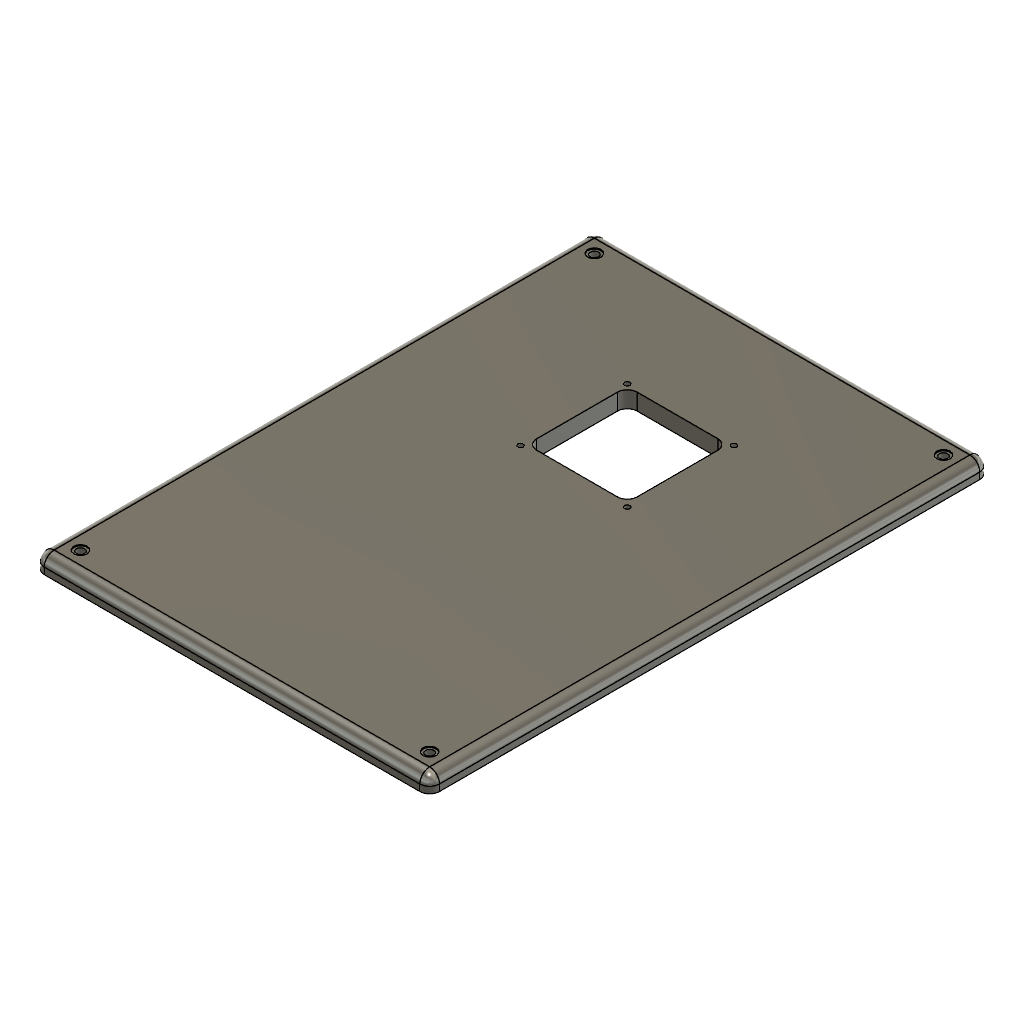
DMX Unit up (Autodesk Fusion 360 design; units mm, degrees)
part number: 2026-09-09-19-26-09-695
Autodesk Fusion 360 part; units mm, degrees
note: some values were not read from the file. Chosen so that the rebuilt part matches the saved one: which face or edge a step refers to; a direction.
(part 1 of 2)
sketch "Esquisse1" plane through (0, 0, 0) normal (0, 1, 0) x (1, 0, 0)
  line L0 (0, 0) -> (120, 0)
  line L1 (120, 0) -> (120, 170)
  line L2 (120, 170) -> (0, 170)
  line L3 (0, 170) -> (0, 0)
  dimension "d1" = 120
  dimension "d2" = 170
  constraint horizontal L0
  constraint vertical L1
  constraint horizontal L2
  constraint vertical L3
  constraint coincident L0.start L3.end
  measures "d1" distance of L0.start L0.end
  measures "d2" distance of L0.end L1.end
sketch "Esquisse2" plane through (0, 100, 0) normal (0, 1, 0) x (1, 0, 0)
  line L0 (5, 165) -> (115, 165)
  line L1 (115, 165) -> (115, 5)
  line L2 (115, 5) -> (5, 5)
  line L3 (5, 5) -> (5, 165)
  line L4 (0, 170) -> (120, 170)
  line L5 (120, 170) -> (120, 0)
  line L6 (120, 0) -> (0, 0)
  line L7 (0, 0) -> (0, 170)
  line L8 (0, 170) -> (0, 0)
  line L9 (0, 0) -> (120, 0)
  line L10 (120, 0) -> (120, 170)
  line L11 (120, 170) -> (0, 170)
  dimension "d5" = 120
  dimension "d6" = 170
  dimension "d7" = 5
  dimension "d8" = 5
  dimension "d9" = 5
  dimension "d10" = 5
  constraint horizontal L0
  constraint vertical L1
  constraint vertical L3
  constraint horizontal L4
  constraint vertical L5
  constraint horizontal L6
  constraint vertical L7
  measures "d5" distance of L4.start L4.end
  measures "d6" distance of L4.end L5.end
  measures "d7" distance of L0 L4
  measures "d8" distance of L3 L7
  measures "d9" distance of L2 L6
  measures "d10" distance of L1 L5
sketch "Esquisse3" plane through (0, 0, 0) normal (0, 0, 1) x (1, 0, 0)
  line L0 (0, 0) -> (120, 0)
  line L1 (120, 0) -> (120, 100)
  line L2 (120, 100) -> (0, 100)
  line L3 (0, 100) -> (0, 0)
  line L4 (0, 100) -> (120, 100)
  line L5 (120, 100) -> (120, 0)
  line L6 (120, 0) -> (0, 0)
  line L7 (0, 0) -> (0, 100)
  circle A0 centre (30, 30) radius 8
  circle A1 centre (90, 30) radius 8
  line L8 (52, 70) -> (68, 70)
  line L9 (68, 70) -> (68, 57)
  line L10 (68, 57) -> (52, 57)
  line L11 (52, 57) -> (52, 70)
  dimension "d13" = 16
  dimension "d14" = 30
  dimension "d15" = 120
  dimension "d16" = 30
  dimension "d17" = 16
  dimension "d18" = 30
  dimension "d19" = 30
  dimension "d20" = 16
  dimension "d21" = 13
  dimension "d22" = 52
  constraint horizontal L4
  constraint vertical L5
  constraint horizontal L6
  constraint vertical L7
  constraint coincident L2.end L3.start
  constraint horizontal L8
  constraint vertical L9
  constraint horizontal L10
  constraint vertical L11
  measures "d13" diameter of A0
  measures "d14" distance of L6 A0.centre
  measures "d15" distance of L0.end L0.start
  measures "d16" distance of L7 A0.centre
  measures "d17" diameter of A1
  measures "d18" distance of L6 A1.centre
  measures "d19" distance of L5 A1.centre
  measures "d20" distance of L8.start L8.end
  measures "d21" distance of L8.end L9.end
  measures "d22" distance of L5 L9
sketch "Esquisse4" plane through (0, 0, 0) normal (0, 0, 1) x (1, 0, 0)
  line L0 (68, 70) -> (68, 57)
  line L1 (68, 57) -> (52, 57)
  line L2 (52, 57) -> (52, 70)
  line L3 (52, 70) -> (68, 70)
  circle A0 centre (30, 30) radius 8
  circle A1 centre (90, 30) radius 8
  line L4 (0, 0) -> (120, 0)
  line L5 (120, 0) -> (120, 100)
  line L6 (120, 100) -> (0, 100)
  line L7 (0, 100) -> (0, 0)
  line L8 (30, 80) -> (90, 80) construction
  line L9 (90, 80) -> (90, 90) construction
  line L10 (90, 90) -> (30, 90) construction
  line L11 (30, 90) -> (30, 80) construction
  dimension "d25" = 10
sketch "Esquisse5" plane through (0, 0, -170) normal (0, 0, -1) x (-1, 0, 0)
  line L0 (-120, 0) -> (0, 0)
  line L1 (0, 0) -> (0, 100)
  line L2 (0, 100) -> (-120, 100)
  line L3 (-120, 100) -> (-120, 0)
  line L4 (-73, 30) -> (-47, 30)
  line L5 (-47, 30) -> (-47, 20)
  line L6 (-47, 20) -> (-73, 20)
  line L7 (-73, 20) -> (-73, 30)
  dimension "d29" = 26
  dimension "d30" = 10
  dimension "d31" = 20
  dimension "d32" = 47
  constraint horizontal L4
  constraint vertical L5
  constraint horizontal L6
  constraint vertical L7
  measures "d29" distance of L4.start L4.end
  measures "d30" distance of L4.end L5.end
  measures "d31" distance of L0 L6
  measures "d32" distance of L1 L5
sketch "Esquisse6" plane through (0, 0, -170) normal (0, 0, -1) x (-1, 0, 0)
  line L0 (-120, 0) -> (0, 0)
  line L1 (0, 0) -> (0, 100)
  line L2 (0, 100) -> (-120, 100)
  line L3 (-120, 100) -> (-120, 0)
  line L4 (-90, 70) -> (-30, 70) construction
  line L5 (-30, 70) -> (-30, 80) construction
  line L6 (-30, 80) -> (-90, 80) construction
  line L7 (-90, 80) -> (-90, 70) construction
  dimension "d35" = 10
sketch "Esquisse7" plane through (0, 0, 0) normal (0, 1, 0) x (1, 0, 0)
  line L0 (-50, 0) -> (-170, 0)
  line L1 (-170, 0) -> (-170, 170)
  line L2 (-170, 170) -> (-50, 170)
  line L3 (-50, 170) -> (-50, 0)
  constraint horizontal L0
  constraint vertical L1
  constraint horizontal L2
  constraint vertical L3
extrude "Extrusion7" add sketch "Esquisse7" along normal blind 5
sketch "Esquisse8" plane through (0, 5, 0) normal (0, 1, 0) x (-1, 0, 0)
  line L0 (50, -170) -> (170, -170)
  line L1 (170, -170) -> (170, 0)
  line L2 (170, 0) -> (50, 0)
  line L3 (50, 0) -> (50, -170)
  line L4 (90, -100) -> (125, -100)
  line L5 (125, -100) -> (125, -135)
  line L6 (125, -135) -> (90, -135)
  line L7 (90, -135) -> (90, -100)
  line L8 (50, 0) -> (170, 0)
  line L9 (170, 0) -> (170, -170)
  line L10 (170, -170) -> (50, -170)
  line L11 (50, -170) -> (50, 0)
  dimension "d41" = 35
  dimension "d42" = 35
  dimension "d43" = 45
  dimension "d44" = 35
  dimension "d45" = 170
  dimension "d46" = 120
  constraint horizontal L4
  constraint vertical L5
  constraint horizontal L6
  constraint vertical L7
  constraint horizontal L8
  constraint vertical L9
  constraint horizontal L10
  constraint vertical L11
  constraint coincident L0.end L1.start
  constraint coincident L2.end L3.start
  measures "d41" distance of L4.start L4.end
  measures "d42" distance of L4.end L5.end
  measures "d43" distance of L1 L5
  measures "d44" distance of L0 L6
  measures "d45" distance of L1.end L0.end
  measures "d46" distance of L2.end L1.end
extrude "Extrusion8" cut sketch "Esquisse8" against normal blind 60 contours L4 L5 L6 L7
fillet "Congé3" radius 3 4 edges at (-110, 5, 0) (-50, 5, -85) (-170, 5, -85) (-110, 5, -170)
sketch "Esquisse9" plane through (0, 0, 0) normal (0, 0, 1) x (1, 0, 0)
  line L0 (117, 3) -> (117, 100)
  line L1 (3, 100) -> (3, 3)
  line L2 (3, 3) -> (117, 3)
  spline S0 degree 3 poles (27.9161, 84.9932) (27.9562, 85.7465) (28.0314, 87.1592) (28.8829, 88.2822) (29.2804, 88.8063) knots 0 0 0 0 0.220424 0.413335 0.413335 0.413335 0.413335
  spline S1 degree 3 poles (29.2804, 88.8063) (29.8033, 89.2037) (30.9218, 90.0539) (32.3299, 90.13) (33.0798, 90.1705) knots 0 0 0 0 0.192622 0.412035 0.412035 0.412035 0.412035
  spline S2 degree 3 poles (33.0798, 90.1705) (33.8439, 90.1336) (35.2646, 90.0651) (36.4015, 89.2205) (36.927, 88.8301) knots 0 0 0 0 0.223535 0.415648 0.415648 0.415648 0.415648
  spline S3 degree 3 poles (36.927, 88.8301) (37.3205, 88.3148) (38.1635, 87.2105) (38.2379, 85.8178) (38.2776, 85.075) knots 0 0 0 0 0.190128 0.407383 0.407383 0.407383 0.407383
  spline S4 degree 3 poles (38.2776, 85.075) (38.2624, 84.5359) (38.2344, 83.5411) (37.8594, 82.6212) (37.6876, 82.1999) knots 0 0 0 0 0.160213 0.295632 0.295632 0.295632 0.295632
  spline S5 degree 3 poles (37.6876, 82.1999) (37.4686, 81.8464) (37.0298, 81.1378) (36.3319, 80.682) (35.9823, 80.4536) knots 0 0 0 0 0.123109 0.246747 0.246747 0.246747 0.246747
  spline S6 degree 3 poles (35.9823, 80.4536) (35.5708, 80.2718) (34.6869, 79.8813) (33.7196, 79.8475) (33.2026, 79.8295) knots 0 0 0 0 0.133717 0.287224 0.287224 0.287224 0.287224
  spline S7 degree 3 poles (33.2026, 79.8295) (32.6811, 79.8436) (31.7167, 79.8698) (30.8161, 80.2115) (30.4025, 80.3683) knots 0 0 0 0 0.155173 0.28695 0.28695 0.28695 0.28695
  spline S8 degree 3 poles (30.4025, 80.3683) (30.0477, 80.5788) (29.3199, 81.0106) (28.8473, 81.7134) (28.605, 82.0737) knots 0 0 0 0 0.122118 0.250545 0.250545 0.250545 0.250545
  spline S9 degree 3 poles (28.605, 82.0737) (28.4043, 82.5044) (27.9739, 83.4282) (27.9362, 84.4485) (27.9161, 84.9932) knots 0 0 0 0 0.14111 0.302672 0.302672 0.302672 0.302672
  line L3 (61.6542, 90) -> (66.7906, 90)
  spline S10 degree 3 poles (66.7906, 90) (67.2965, 89.9827) (68.214, 89.9514) (68.9666, 89.4341) (69.3042, 89.2019) knots 0 0 0 0 0.148093 0.268627 0.268627 0.268627 0.268627
  spline S11 degree 3 poles (69.3042, 89.2019) (69.5476, 88.8929) (70.0702, 88.2295) (70.1156, 87.3827) (70.1398, 86.9304) knots 0 0 0 0 0.115225 0.247344 0.247344 0.247344 0.247344
  spline S12 degree 3 poles (70.1398, 86.9304) (70.1109, 86.4621) (70.0561, 85.574) (69.4946, 84.8878) (69.2292, 84.5634) knots 0 0 0 0 0.136799 0.259393 0.259393 0.259393 0.259393
  spline S13 degree 3 poles (69.2292, 84.5634) (68.8572, 84.3155) (68.0209, 83.7581) (67.0105, 83.7277) (66.4495, 83.7108) knots 0 0 0 0 0.131606 0.295937 0.295937 0.295937 0.295937
  line L4 (66.4495, 83.7108) -> (64.7578, 83.7108)
  line L5 (64.7578, 83.7108) -> (64.7578, 80)
  line L6 (64.7578, 80) -> (61.6542, 80)
  line L7 (61.6542, 80) -> (61.6542, 90)
  line L8 (78.264, 90) -> (81.3472, 90)
  line L9 (81.3472, 90) -> (81.3472, 84.0421)
  spline S14 degree 3 poles (81.3472, 84.0421) (81.3364, 83.753) (81.3152, 83.1834) (81.1515, 82.6375) (81.0709, 82.3687) knots 0 0 0 0 0.086419 0.170224 0.170224 0.170224 0.170224
  spline S15 degree 3 poles (81.0709, 82.3687) (80.9658, 82.1145) (80.7555, 81.6061) (80.3883, 81.1965) (80.2046, 80.9917) knots 0 0 0 0 0.081874 0.163736 0.163736 0.163736 0.163736
  spline S16 degree 3 poles (80.2046, 80.9917) (80.0113, 80.812) (79.6427, 80.4693) (79.1845, 80.2621) (78.9666, 80.1635) knots 0 0 0 0 0.078572 0.149835 0.149835 0.149835 0.149835
  spline S17 degree 3 poles (78.9666, 80.1635) (78.6385, 80.0662) (77.9335, 79.8571) (77.1977, 79.8391) (76.8042, 79.8295) knots 0 0 0 0 0.102197 0.21965 0.21965 0.21965 0.21965
  spline S18 degree 3 poles (76.8042, 79.8295) (76.5496, 79.8344) (76.0172, 79.8448) (75.4877, 79.9019) (75.2115, 79.9317) knots 0 0 0 0 0.076356 0.159674 0.159674 0.159674 0.159674
  spline S19 degree 3 poles (75.2115, 79.9317) (74.9438, 79.9701) (74.4446, 80.0416) (73.9829, 80.2436) (73.7688, 80.3373) knots 0 0 0 0 0.080667 0.150474 0.150474 0.150474 0.150474
  spline S20 degree 3 poles (73.7688, 80.3373) (73.5773, 80.4518) (73.1823, 80.688) (72.8693, 81.0256) (72.7081, 81.1996) knots 0 0 0 0 0.066557 0.13732 0.13732 0.13732 0.13732
  spline S21 degree 3 poles (72.7081, 81.1996) (72.5619, 81.3825) (72.2822, 81.7325) (72.1249, 82.1515) (72.0498, 82.3516) knots 0 0 0 0 0.069719 0.13342 0.13342 0.13342 0.13342
  spline S22 degree 3 poles (72.0498, 82.3516) (71.9664, 82.6496) (71.8114, 83.2034) (71.7785, 83.7772) (71.7633, 84.0421) knots 0 0 0 0 0.09251 0.171904 0.171904 0.171904 0.171904
  line L10 (71.7633, 84.0421) -> (71.7633, 90)
  line L11 (71.7633, 90) -> (74.8465, 90)
  line L12 (74.8465, 90) -> (74.8465, 83.9003)
  spline S23 degree 3 poles (74.8465, 83.9003) (74.8599, 83.6484) (74.8851, 83.1758) (75.168, 82.7986) (75.3001, 82.6224) knots 0 0 0 0 0.073721 0.138349 0.138349 0.138349 0.138349
  spline S24 degree 3 poles (75.3001, 82.6224) (75.4734, 82.4883) (75.8426, 82.2027) (76.3104, 82.1763) (76.5587, 82.1623) knots 0 0 0 0 0.064202 0.136827 0.136827 0.136827 0.136827
  spline S25 degree 3 poles (76.5587, 82.1623) (76.805, 82.1762) (77.2693, 82.2022) (77.6375, 82.4835) (77.8104, 82.6156) knots 0 0 0 0 0.072093 0.135879 0.135879 0.135879 0.135879
  spline S26 degree 3 poles (77.8104, 82.6156) (77.9425, 82.7913) (78.2274, 83.1701) (78.2512, 83.6454) (78.264, 83.9003) knots 0 0 0 0 0.064484 0.139042 0.139042 0.139042 0.139042
  line L13 (78.264, 83.9003) -> (78.264, 90)
  line L14 (82.691, 90) -> (92.0839, 90)
  line L15 (92.0839, 90) -> (92.0839, 87.5307)
  line L16 (92.0839, 87.5307) -> (88.9325, 87.5307)
  line L17 (88.9325, 87.5307) -> (88.9325, 80)
  line L18 (88.9325, 80) -> (85.8424, 80)
  line L19 (85.8424, 80) -> (85.8424, 87.5307)
  line L20 (85.8424, 87.5307) -> (82.691, 87.5307)
  line L21 (82.691, 87.5307) -> (82.691, 90)
  line L22 (46.4495, 90) -> (49.5327, 90)
  line L23 (49.5327, 90) -> (49.5327, 84.0421)
  spline S27 degree 3 poles (49.5327, 84.0421) (49.522, 83.753) (49.5007, 83.1834) (49.3371, 82.6375) (49.2565, 82.3687) knots 0 0 0 0 0.086419 0.170223 0.170223 0.170223 0.170223
  spline S28 degree 3 poles (49.2565, 82.3687) (49.1513, 82.1145) (48.941, 81.6061) (48.5738, 81.1965) (48.3902, 80.9917) knots 0 0 0 0 0.081874 0.163737 0.163737 0.163737 0.163737
  spline S29 degree 3 poles (48.3902, 80.9917) (48.1969, 80.812) (47.8283, 80.4693) (47.37, 80.2621) (47.1521, 80.1635) knots 0 0 0 0 0.078572 0.149834 0.149834 0.149834 0.149834
  spline S30 degree 3 poles (47.1521, 80.1635) (46.8241, 80.0662) (46.119, 79.8571) (45.3832, 79.8391) (44.9898, 79.8295) knots 0 0 0 0 0.102197 0.21965 0.21965 0.21965 0.21965
  spline S31 degree 3 poles (44.9898, 79.8295) (44.7352, 79.8344) (44.2028, 79.8448) (43.6733, 79.9019) (43.397, 79.9317) knots 0 0 0 0 0.076356 0.159673 0.159673 0.159673 0.159673
  spline S32 degree 3 poles (43.397, 79.9317) (43.1294, 79.9701) (42.6301, 80.0416) (42.1685, 80.2436) (41.9543, 80.3373) knots 0 0 0 0 0.080667 0.150474 0.150474 0.150474 0.150474
  spline S33 degree 3 poles (41.9543, 80.3373) (41.7628, 80.4518) (41.3678, 80.688) (41.0549, 81.0256) (40.8936, 81.1996) knots 0 0 0 0 0.066557 0.13732 0.13732 0.13732 0.13732
  spline S34 degree 3 poles (40.8936, 81.1996) (40.7474, 81.3825) (40.4678, 81.7325) (40.3105, 82.1515) (40.2353, 82.3516) knots 0 0 0 0 0.069719 0.13342 0.13342 0.13342 0.13342
  spline S35 degree 3 poles (40.2353, 82.3516) (40.1519, 82.6496) (39.9969, 83.2034) (39.964, 83.7772) (39.9488, 84.0421) knots 0 0 0 0 0.09251 0.171904 0.171904 0.171904 0.171904
  line L24 (39.9488, 84.0421) -> (39.9488, 90)
  line L25 (39.9488, 90) -> (43.0321, 90)
  line L26 (43.0321, 90) -> (43.0321, 83.9003)
  spline S36 degree 3 poles (43.0321, 83.9003) (43.0455, 83.6484) (43.0706, 83.1758) (43.3535, 82.7986) (43.4857, 82.6224) knots 0 0 0 0 0.073721 0.138349 0.138349 0.138349 0.138349
  spline S37 degree 3 poles (43.4857, 82.6224) (43.6589, 82.4883) (44.0281, 82.2027) (44.4959, 82.1763) (44.7442, 82.1623) knots 0 0 0 0 0.064202 0.136827 0.136827 0.136827 0.136827
  spline S38 degree 3 poles (44.7442, 82.1623) (44.9905, 82.1762) (45.4548, 82.2022) (45.8231, 82.4835) (45.9959, 82.6156) knots 0 0 0 0 0.072093 0.135879 0.135879 0.135879 0.135879
  spline S39 degree 3 poles (45.9959, 82.6156) (46.128, 82.7913) (46.4129, 83.1701) (46.4367, 83.6454) (46.4495, 83.9003) knots 0 0 0 0 0.064484 0.139042 0.139042 0.139042 0.139042
  line L27 (46.4495, 83.9003) -> (46.4495, 90)
  line L28 (50.8765, 90) -> (60.2694, 90)
  line L29 (60.2694, 90) -> (60.2694, 87.5307)
  line L30 (60.2694, 87.5307) -> (57.118, 87.5307)
  line L31 (57.118, 87.5307) -> (57.118, 80)
  line L32 (57.118, 80) -> (54.028, 80)
  line L33 (54.028, 80) -> (54.028, 87.5307)
  line L34 (54.028, 87.5307) -> (50.8765, 87.5307)
  line L35 (50.8765, 87.5307) -> (50.8765, 90)
  line L36 (3, 100) -> (117, 100)
  line L37 (117, 100) -> (117, 3)
  line L38 (117, 3) -> (3, 3)
  line L39 (3, 3) -> (3, 100)
  circle A0 centre (33, 28) radius 12
  circle A1 centre (87, 28) radius 12
  line L40 (42.5, 28) -> (23.5, 28) construction
  line L41 (60, 131) -> (60, -75) construction
  line L42 (23.5, 16) -> (23.5, 40) construction
  circle A2 centre (23.5, 40) radius 1.75
  line L43 (23.5, 28) -> (42.5, 28) construction
  line L44 (42.5, 40) -> (42.5, 16) construction
  circle A3 centre (42.5, 16) radius 1.75
  line L45 (96.5, 28) -> (77.5, 28) construction
  line L46 (77.5, 16) -> (77.5, 40) construction
  circle A4 centre (77.5, 40) radius 1.75
  line L47 (96.5, 40) -> (96.5, 16) construction
  circle A5 centre (96.5, 16) radius 1.75
  line L48 (117, 100) -> (3, 100)
  line L49 (51.95, 57) -> (68.05, 57)
  line L50 (68.05, 57) -> (68.05, 70.5)
  line L51 (68.05, 70.5) -> (51.95, 70.5)
  line L52 (51.95, 70.5) -> (51.95, 57)
  point P0 (33, 28)
  point P1 (33, 28)
  point P2 (33, 28)
  point P3 (87, 28)
  dimension "d55" = 114
  dimension "d56" = 97
  dimension "d59" = 24
  dimension "d60" = 24
  dimension "d61" = 25
  dimension "d62" = 25
  dimension "d63" = 30
  dimension "d64" = 30
  dimension "d69" = 19
  dimension "d70" = 24
  dimension "d71" = 3.5
  dimension "d72" = 19
  dimension "d73" = 24
  dimension "d74" = 3.5
  dimension "d75" = 19
  dimension "d76" = 24
  dimension "d77" = 3.5
  dimension "d78" = 24
  dimension "d79" = 3.5
  dimension "d134" = 13.5
  dimension "d135" = 16.1
  dimension "d136" = 48.95
  dimension "d137" = 48.95
  constraint horizontal L36
  constraint vertical L37
  constraint horizontal L38
  constraint vertical L39
  constraint coincident L0.start L2.end
  constraint coincident L1.start L36.start
  constraint midpoint L40 P2
  constraint coincident P2 P1
  constraint perpendicular L39 L40
  constraint perpendicular L2 L41
  constraint midpoint L40.end L42
  constraint perpendicular L40 L42
  constraint coincident L42.end A2.centre
  constraint midpoint L43 P2
  constraint parallel L40 L43
  constraint midpoint L40.start L44
  constraint perpendicular L43 L44
  constraint coincident L44.end A3.centre
  constraint midpoint L45 P3
  constraint coincident P3 A1.centre
  constraint horizontal L45
  constraint midpoint L45.end L46
  constraint perpendicular L45 L46
  constraint coincident L46.end A4.centre
  constraint midpoint L45.start L47
  constraint perpendicular L45 L47
  constraint coincident L47.end A5.centre
  constraint horizontal L49
  constraint vertical L50
  constraint horizontal L51
  constraint vertical L52
  measures "d55" distance of L1.start L0.end
  measures "d56" distance of L0.end L0.start
  measures "d59" diameter of A0
  measures "d60" diameter of A1
  measures "d61" distance of L38 P3
  measures "d62" distance of L38 P2
  measures "d63" distance of L37 P3
  measures "d64" distance of L39 P2
  measures "d69" distance of L40.start L40.end
  measures "d70" distance of L42.start L42.end
  measures "d71" diameter of A2
  measures "d72" distance of L40.end L40.start
  measures "d73" distance of L44.start L44.end
  measures "d74" diameter of A3
  measures "d75" distance of L45.start L45.end
  measures "d76" distance of L46.start L46.end
  measures "d77" diameter of A4
  measures "d78" distance of L47.start L47.end
  measures "d79" diameter of A5
  measures "d134" distance of L49.start L51.end
  measures "d135" distance of L49.start L49.end
  measures "d136" distance of L37 L50
  measures "d137" distance of L39 L52
extrude "Extrusion9" cut sketch "Esquisse9" against normal blind 20 contours A0 | A1 | A2 | A3 | A4 | A5
sketch "Esquisse10" plane through (0, 0, 0) normal (0, 1, 0) x (1, 0, 0)
sketch "Esquisse11" plane through (0, 10, 0) normal (0, 1, 0) x (-1, 0, 0)
  line L0 (-5, -5) -> (-115, -5)
  line L1 (-115, -5) -> (-115, -165)
  line L2 (-115, -165) -> (-5, -165)
  line L3 (-5, -165) -> (-5, -5)
  line L4 (-5, -165) -> (-13, -165)
  line L5 (-13, -165) -> (-13, -157)
  line L6 (-13, -157) -> (-5, -157)
  line L7 (-5, -157) -> (-5, -165)
  line L8 (-115, -165) -> (-107, -165)
  line L9 (-107, -165) -> (-107, -157)
  line L10 (-107, -157) -> (-115, -157)
  line L11 (-115, -157) -> (-115, -165)
  line L12 (-115, -5) -> (-107, -5)
  line L13 (-107, -5) -> (-107, -13)
  line L14 (-107, -13) -> (-115, -13)
  line L15 (-115, -13) -> (-115, -5)
  line L16 (-5, -5) -> (-13, -5)
  line L17 (-13, -5) -> (-13, -13)
  line L18 (-13, -13) -> (-5, -13)
  line L19 (-5, -13) -> (-5, -5)
  constraint horizontal L4
  constraint vertical L5
  constraint horizontal L6
  constraint vertical L7
  constraint coincident L2.end L3.start
  constraint horizontal L8
  constraint vertical L9
  constraint horizontal L10
  constraint vertical L11
  constraint coincident L1.end L2.start
  constraint horizontal L12
  constraint vertical L13
  constraint horizontal L14
  constraint vertical L15
  constraint coincident L0.end L1.start
  constraint horizontal L16
  constraint vertical L17
  constraint horizontal L18
  constraint vertical L19
  constraint coincident L0.start L3.end
sketch "Esquisse12" plane through (0, 5, 0) normal (0, 1, 0) x (-1, 0, 0)
  line L0 (125, -100) -> (125, -135)
  line L1 (125, -135) -> (90, -135)
  line L2 (90, -135) -> (90, -100)
  line L3 (90, -100) -> (125, -100)
  line L4 (53, -167) -> (167, -167)
  line L5 (167, -167) -> (167, -3)
  line L6 (167, -3) -> (53, -3)
  line L7 (53, -3) -> (53, -167)
  circle A0 centre (163, -163) radius 1.25
  circle A1 centre (57, -163) radius 1.25
  circle A2 centre (57, -7) radius 1.25
  circle A3 centre (163, -7) radius 1.25
  dimension "d86" = 2.5
  dimension "d87" = 4
  dimension "d88" = 4
  dimension "d89" = 2.5
  dimension "d90" = 4
  dimension "d91" = 4
  dimension "d92" = 2.5
  dimension "d93" = 2.5
  dimension "d94" = 4
  dimension "d95" = 4
  dimension "d96" = 4
  dimension "d97" = 4
  measures "d86" diameter of A0
  measures "d87" distance of L4 A0.centre
  measures "d88" distance of L5 A0.centre
  measures "d89" diameter of A1
  measures "d90" distance of L4 A1.centre
  measures "d91" distance of L7 A1.centre
  measures "d92" diameter of A3
  measures "d93" diameter of A2
  measures "d94" distance of L7 A2.centre
  measures "d95" distance of L6 A2.centre
  measures "d96" distance of L6 A3.centre
  measures "d97" distance of L5 A3.centre
extrude "Extrusion11" cut sketch "Esquisse12" against normal blind 60 contours A0 | A1 | A2 | A3
sketch "Esquisse13" plane through (0, 0, -165) normal (0, 0, 1) x (1, 0, 0)
  line L0 (13, 100) -> (13, 10)
  line L1 (13, 10) -> (107, 10)
  line L2 (107, 10) -> (107, 100)
  line L3 (107, 100) -> (13, 100)
sketch "Esquisse14" plane through (0, 0, -170) normal (0, 0, -1) x (-1, 0, 0)
  line L0 (-66.7462, 80) -> (-61.6098, 80)
  spline S0 degree 3 poles (-61.6098, 80) (-61.104, 79.9827) (-60.1864, 79.9514) (-59.4338, 79.4341) (-59.0962, 79.2019) knots 0 0 0 0 0.148093 0.268627 0.268627 0.268627 0.268627
  spline S1 degree 3 poles (-59.0962, 79.2019) (-58.8528, 78.8929) (-58.3302, 78.2295) (-58.2848, 77.3827) (-58.2606, 76.9304) knots 0 0 0 0 0.115225 0.247344 0.247344 0.247344 0.247344
  spline S2 degree 3 poles (-58.2606, 76.9304) (-58.2895, 76.4621) (-58.3443, 75.574) (-58.9058, 74.8878) (-59.1712, 74.5634) knots 0 0 0 0 0.136799 0.259393 0.259393 0.259393 0.259393
  spline S3 degree 3 poles (-59.1712, 74.5634) (-59.5432, 74.3155) (-60.3795, 73.7581) (-61.3899, 73.7277) (-61.9509, 73.7108) knots 0 0 0 0 0.131606 0.295938 0.295938 0.295938 0.295938
  line L1 (-61.9509, 73.7108) -> (-63.6426, 73.7108)
  line L2 (-63.6426, 73.7108) -> (-63.6426, 70)
  line L3 (-63.6426, 70) -> (-66.7462, 70)
  line L4 (-66.7462, 70) -> (-66.7462, 80)
  line L5 (-78.3492, 80) -> (-75.4638, 80)
  line L6 (-75.4638, 80) -> (-71.6985, 74.4675)
  line L7 (-71.6985, 74.4675) -> (-71.6985, 80)
  line L8 (-71.6985, 80) -> (-68.7858, 80)
  line L9 (-68.7858, 80) -> (-68.7858, 70)
  line L10 (-68.7858, 70) -> (-71.6985, 70)
  line L11 (-71.6985, 70) -> (-75.4434, 75.4907)
  line L12 (-75.4434, 75.4907) -> (-75.4434, 70)
  line L13 (-75.4434, 70) -> (-78.3492, 70)
  line L14 (-78.3492, 70) -> (-78.3492, 80)
  line L15 (-117, 100) -> (-117, 3)
  line L16 (-117, 3) -> (-3, 3)
  line L17 (-3, 3) -> (-3, 100)
  line L18 (-3, 100) -> (-117, 100)
  line L19 (-50.1364, 80) -> (-47.0532, 80)
  line L20 (-47.0532, 80) -> (-47.0532, 74.0421)
  spline S4 degree 3 poles (-47.0532, 74.0421) (-47.064, 73.753) (-47.0852, 73.1834) (-47.2489, 72.6375) (-47.3295, 72.3687) knots 0 0 0 0 0.086419 0.170223 0.170223 0.170223 0.170223
  spline S5 degree 3 poles (-47.3295, 72.3687) (-47.4346, 72.1145) (-47.6449, 71.6061) (-48.0122, 71.1965) (-48.1958, 70.9917) knots 0 0 0 0 0.081874 0.163737 0.163737 0.163737 0.163737
  spline S6 degree 3 poles (-48.1958, 70.9917) (-48.3891, 70.812) (-48.7577, 70.4693) (-49.2159, 70.2621) (-49.4338, 70.1635) knots 0 0 0 0 0.078572 0.149834 0.149834 0.149834 0.149834
  spline S7 degree 3 poles (-49.4338, 70.1635) (-49.7619, 70.0662) (-50.4669, 69.8571) (-51.2027, 69.8391) (-51.5962, 69.8295) knots 0 0 0 0 0.102197 0.21965 0.21965 0.21965 0.21965
  spline S8 degree 3 poles (-51.5962, 69.8295) (-51.8508, 69.8344) (-52.3832, 69.8448) (-52.9127, 69.9019) (-53.189, 69.9317) knots 0 0 0 0 0.076356 0.159674 0.159674 0.159674 0.159674
  spline S9 degree 3 poles (-53.189, 69.9317) (-53.4566, 69.9701) (-53.9558, 70.0416) (-54.4175, 70.2436) (-54.6317, 70.3373) knots 0 0 0 0 0.080667 0.150474 0.150474 0.150474 0.150474
  spline S10 degree 3 poles (-54.6317, 70.3373) (-54.8231, 70.4518) (-55.2181, 70.688) (-55.5311, 71.0256) (-55.6924, 71.1996) knots 0 0 0 0 0.066557 0.137321 0.137321 0.137321 0.137321
  spline S11 degree 3 poles (-55.6924, 71.1996) (-55.8385, 71.3825) (-56.1182, 71.7325) (-56.2755, 72.1515) (-56.3506, 72.3516) knots 0 0 0 0 0.069719 0.13342 0.13342 0.13342 0.13342
  spline S12 degree 3 poles (-56.3506, 72.3516) (-56.434, 72.6496) (-56.589, 73.2034) (-56.6219, 73.7772) (-56.6371, 74.0421) knots 0 0 0 0 0.09251 0.171904 0.171904 0.171904 0.171904
  line L21 (-56.6371, 74.0421) -> (-56.6371, 80)
  line L22 (-56.6371, 80) -> (-53.5539, 80)
  line L23 (-53.5539, 80) -> (-53.5539, 73.9003)
  spline S13 degree 3 poles (-53.5539, 73.9003) (-53.5405, 73.6484) (-53.5153, 73.1758) (-53.2324, 72.7986) (-53.1003, 72.6224) knots 0 0 0 0 0.073721 0.138349 0.138349 0.138349 0.138349
  spline S14 degree 3 poles (-53.1003, 72.6224) (-52.927, 72.4883) (-52.5578, 72.2027) (-52.09, 72.1763) (-51.8417, 72.1623) knots 0 0 0 0 0.064202 0.136827 0.136827 0.136827 0.136827
  spline S15 degree 3 poles (-51.8417, 72.1623) (-51.5954, 72.1762) (-51.1311, 72.2022) (-50.7629, 72.4835) (-50.59, 72.6156) knots 0 0 0 0 0.072094 0.135879 0.135879 0.135879 0.135879
  spline S16 degree 3 poles (-50.59, 72.6156) (-50.4579, 72.7913) (-50.173, 73.1701) (-50.1492, 73.6454) (-50.1364, 73.9003) knots 0 0 0 0 0.064484 0.139042 0.139042 0.139042 0.139042
  line L24 (-50.1364, 73.9003) -> (-50.1364, 80)
  line L25 (-45.7094, 80) -> (-36.3165, 80)
  line L26 (-36.3165, 80) -> (-36.3165, 77.5307)
  line L27 (-36.3165, 77.5307) -> (-39.4679, 77.5307)
  line L28 (-39.4679, 77.5307) -> (-39.4679, 70)
  line L29 (-39.4679, 70) -> (-42.558, 70)
  line L30 (-42.558, 70) -> (-42.558, 77.5307)
  line L31 (-42.558, 77.5307) -> (-45.7094, 77.5307)
  line L32 (-45.7094, 77.5307) -> (-45.7094, 80)
  line L33 (-83.6835, 80) -> (-80.5866, 80)
  line L34 (-80.5866, 80) -> (-80.5866, 70)
  line L35 (-80.5866, 70) -> (-83.6835, 70)
  line L36 (-83.6835, 70) -> (-83.6835, 80)
  line L37 (-73, 49.0881) -> (-47, 49.0881)
  line L38 (-47, 49.0881) -> (-47, 39.0881)
  line L39 (-47, 39.0881) -> (-73, 39.0881)
  line L40 (-73, 39.0881) -> (-73, 49.0881)
  dimension "d100" = 26
  dimension "d101" = 10
  dimension "d102" = 44
  dimension "d103" = 44
  constraint horizontal L37
  constraint vertical L38
  constraint horizontal L39
  constraint vertical L40
  measures "d100" distance of L37.start L37.end
  measures "d101" distance of L37.end L38.end
  measures "d102" distance of L17 L38
  measures "d103" distance of L15 L40
extrude "Extrusion12" cut sketch "Esquisse14" against normal blind 20.338 contours L37 L38 L39 L40
sketch "Esquisse15" plane through (5, 0, 0) normal (1, 0, 0) x (0, 0, -1)
  line L0 (13, 100) -> (13, 10)
  line L1 (13, 10) -> (157, 10)
  line L2 (157, 10) -> (157, 100)
  line L3 (157, 100) -> (13, 100)
sketch "Esquisse16" plane through (0, 100, 0) normal (0, 1, 0) x (-1, 0, 0)
  line L0 (-107, -13) -> (-107, -5)
  line L1 (-13, -5) -> (-13, -13)
  line L2 (-13, -13) -> (-5, -13)
  line L3 (-5, -157) -> (-13, -157)
  line L4 (-13, -157) -> (-13, -165)
  line L5 (-107, -165) -> (-107, -157)
  line L6 (-107, -157) -> (-115, -157)
  line L7 (-115, -13) -> (-107, -13)
  circle A0 centre (-114.25, -5.75) radius 1.6
  circle A1 centre (163, -7) radius 1.25
  circle A2 centre (-5.75, -5.75) radius 1.6
  line L8 (-120, 0) -> (0, 0)
  line L9 (0, 0) -> (0, -170)
  line L10 (0, -170) -> (-120, -170)
  line L11 (-120, -170) -> (-120, 0)
  line L12 (-120, 0) -> (-120, -85)
  line L13 (-120, -85) -> (0, -85)
  circle A3 centre (-5.75, -164.25) radius 1.6
  circle A4 centre (-114.25, -164.25) radius 1.6
  circle A5 centre (57, -7) radius 2
  circle A6 centre (163, -7) radius 2
  circle A7 centre (57, -163) radius 2
  circle A8 centre (163, -163) radius 2
  line L14 (-107, -5) -> (-115, -5)
  line L15 (-115, -5) -> (-115, -13)
  line L16 (-5, -13) -> (-5, -5)
  line L17 (-5, -5) -> (-13, -5)
  line L18 (-13, -165) -> (-5, -165)
  line L19 (-5, -165) -> (-5, -157)
  line L20 (-115, -157) -> (-115, -165)
  line L21 (-115, -165) -> (-107, -165)
  dimension "d108" = 3.2
  dimension "d109" = 2.5
  dimension "d110" = 3.2
  dimension "d113" = 170
  dimension "d114" = 4
  dimension "d115" = 4
  dimension "d116" = 4
  constraint horizontal L8
  constraint vertical L9
  constraint horizontal L10
  constraint vertical L11
  constraint midpoint L9 L13.end
  constraint perpendicular L9 L13
  constraint symmetric A0 L13 A4
  constraint symmetric A2 L13 A3
  constraint concentric A1 A6
  measures "d108" diameter of A0
  measures "d109" diameter of A1
  measures "d110" diameter of A2
  measures "d113" distance of L8.start L10.end
  measures "d114" diameter of A6
  measures "d115" diameter of A7
  measures "d116" diameter of A8
extrude "Extrusion13" cut sketch "Esquisse16" against normal blind 5 contours A0 L14 L15 | A0 L14 L15 | A2 L16 L17 | A2 L16 L17 | A3 L18 L19 | A3 L18 L19 | A4 L20 L21 | A4 L20 L21
extrude "Extrusion14" cut sketch "Esquisse16" against normal blind 0.3 from surface at -95 contours A5 | A6 | A7 | A8
sketch "Esquisse17" plane through (0, 10, 0) normal (0, 1, 0) x (-1, 0, 0)
  line L0 (-13, -11.5) -> (-13, -5)
  line L1 (-13, -5) -> (-107, -5)
  line L2 (-107, -5) -> (-107, -11.5)
  arc A0 (-108.5, -13) -> (-107, -11.5) centre (-108.5, -11.5) ccw
  line L3 (-108.5, -13) -> (-115, -13)
  line L4 (-115, -13) -> (-115, -157)
  line L5 (-115, -157) -> (-108.5, -157)
  arc A1 (-107, -158.5) -> (-108.5, -157) centre (-108.5, -158.5) ccw
  line L6 (-107, -158.5) -> (-107, -165)
  line L7 (-107, -165) -> (-13, -165)
  line L8 (-13, -165) -> (-13, -158.5)
  arc A2 (-11.5, -157) -> (-13, -158.5) centre (-11.5, -158.5) ccw
  line L9 (-11.5, -157) -> (-5, -157)
  line L10 (-5, -157) -> (-5, -13)
  line L11 (-5, -13) -> (-11.5, -13)
  arc A3 (-13, -11.5) -> (-11.5, -13) centre (-11.5, -11.5) ccw
  line L12 (-23, -60) -> (-41, -60)
  line L13 (-41, -60) -> (-41, -30)
  line L14 (-41, -30) -> (-23, -30)
  line L15 (-23, -30) -> (-23, -60)
  line L16 (-25, -60) -> (-39, -60)
  line L17 (-39, -60) -> (-39, -30)
  line L18 (-39, -30) -> (-25, -30)
  line L19 (-25, -30) -> (-25, -60)
  line L20 (-5, -157) -> (-5, -13)
  line L21 (0, -15) -> (-120, -15)
  line L22 (-120, -15) -> (-60, -15)
  line L23 (-60, -15) -> (-60, -165)
  line L24 (-97, -30) -> (-97, -60)
  line L25 (-95, -30) -> (-95, -60)
  line L26 (-81, -60) -> (-81, -30)
  line L27 (-79, -60) -> (-79, -30)
  line L28 (-97, -60) -> (-79, -60)
  line L29 (-79, -30) -> (-97, -30)
  dimension "d122" = 2
  dimension "d123" = 2
  dimension "d124" = 18
  dimension "d125" = 18
  constraint horizontal L12
  constraint vertical L13
  constraint horizontal L14
  constraint vertical L15
  constraint horizontal L16
  constraint vertical L17
  constraint horizontal L18
  constraint vertical L19
  constraint coincident L14 L17.end
  constraint coincident L12 L16.start
  constraint perpendicular L4 L21
  constraint midpoint L21 L22.end
  constraint perpendicular L22 L23
  constraint symmetric L12.start L23 L24.end
  constraint symmetric L12.end L23 L27.start
  constraint symmetric L13.end L23 L27.end
  constraint symmetric L14.end L23 L24.start
  constraint symmetric L16.start L23 L25.end
  constraint symmetric L16.end L23 L26.start
  constraint symmetric L17.end L23 L26.end
  constraint symmetric L18.end L23 L25.start
  measures "d122" distance of L15 L19
  measures "d123" distance of L13 L17
  measures "d124" distance of L12.start L12.end
  measures "d125" distance of L15 L20
sketch "Esquisse18" plane through (0, 0, -30) normal (0, 0, 1) x (1, 0, 0)
  line L0 (97, 10) -> (97, 24)
  line L1 (97, 24) -> (95, 24)
  line L2 (95, 24) -> (95, 10)
  line L3 (81, 10) -> (81, 24)
  line L4 (81, 24) -> (79, 24)
  line L5 (79, 24) -> (79, 10)
  line L6 (95, 24) -> (95, 10)
  line L7 (95, 24) -> (97, 24)
  line L8 (97, 24) -> (97, 25)
  line L9 (97, 25) -> (95, 25)
  line L10 (95, 25) -> (95, 24)
  line L11 (79, 24) -> (81, 24)
  line L12 (81, 24) -> (81, 25)
  line L13 (81, 25) -> (79, 25)
  line L14 (79, 25) -> (79, 24)
  line L15 (23, 25) -> (25, 25)
  line L16 (25, 25) -> (25, 24)
  line L17 (25, 24) -> (23, 24)
  line L18 (23, 24) -> (23, 25)
  line L19 (39, 25) -> (41, 25)
  line L20 (41, 25) -> (41, 24)
  line L21 (41, 24) -> (39, 24)
  line L22 (39, 24) -> (39, 25)
  circle A0 centre (95, 24.5) radius 0.5
  circle A1 centre (81, 24.5) radius 0.5
  circle A2 centre (25, 24.5) radius 0.5
  circle A3 centre (39, 24.5) radius 0.5
  line L23 (80.5, 24) -> (81, 24)
  line L24 (81, 24) -> (81, 10)
  line L25 (81, 10) -> (80.5, 10)
  line L26 (80.5, 10) -> (80.5, 24)
  line L27 (95, 24) -> (95.5, 24)
  line L28 (95.5, 24) -> (95.5, 22)
  line L29 (95.5, 22) -> (95, 22)
  line L30 (95, 22) -> (95, 24)
  line L31 (25, 24) -> (24.5, 24)
  line L32 (24.5, 24) -> (24.5, 22)
  line L33 (24.5, 22) -> (25, 22)
  line L34 (25, 22) -> (25, 24)
  line L35 (39, 24) -> (39.5, 24)
  line L36 (39.5, 24) -> (39.5, 22)
  line L37 (39.5, 22) -> (39, 22)
  line L38 (39, 22) -> (39, 24)
  line L39 (79, 10) -> (81, 10)
  line L40 (95, 10) -> (97, 10)
  constraint coincident L1.end L2.start
  constraint coincident L2.end L6.end
  constraint horizontal L7
  constraint vertical L8
  constraint horizontal L9
  constraint vertical L10
  constraint horizontal L11
  constraint vertical L12
  constraint horizontal L13
  constraint vertical L14
  constraint coincident L4.end L5.start
  constraint horizontal L15
  constraint vertical L16
  constraint horizontal L17
  constraint vertical L18
  constraint horizontal L19
  constraint vertical L20
  constraint horizontal L21
  constraint vertical L22
  constraint midpoint L10 A0.centre
  constraint coincident L9.end A0
  constraint midpoint L12 A1.centre
  constraint coincident L12.end A1
  constraint midpoint L16 A2.centre
  constraint coincident L15.end A2
  constraint midpoint L22 A3.centre
  constraint coincident L19.start A3
  constraint horizontal L23
  constraint vertical L24
  constraint horizontal L25
  constraint vertical L26
  constraint coincident L3.start L24.end
  constraint coincident L4 L23.start
  constraint horizontal L27
  constraint vertical L28
  constraint horizontal L29
  constraint vertical L30
  constraint horizontal L31
  constraint vertical L32
  constraint horizontal L33
  constraint vertical L34
  constraint horizontal L35
  constraint vertical L36
  constraint horizontal L37
  constraint vertical L38
sketch "Esquisse19" plane through (0, 10, 0) normal (0, 1, 0) x (-1, 0, 0)
  line L0 (-97, -30) -> (-79, -30)
  line L1 (-79, -30) -> (-79, -60)
  line L2 (-79, -60) -> (-97, -60)
  line L3 (-97, -60) -> (-97, -30)
  line L4 (-41, -30) -> (-23, -30)
  line L5 (-23, -30) -> (-23, -60)
  line L6 (-23, -60) -> (-41, -60)
  line L7 (-41, -60) -> (-41, -30)
  line L8 (-13, -11.5) -> (-13, -5)
  line L9 (-13, -5) -> (-107, -5)
  line L10 (-107, -5) -> (-107, -11.5)
  arc A0 (-108.5, -13) -> (-107, -11.5) centre (-108.5, -11.5) ccw
  line L11 (-108.5, -13) -> (-115, -13)
  line L12 (-115, -13) -> (-115, -157)
  line L13 (-115, -157) -> (-108.5, -157)
  arc A1 (-107, -158.5) -> (-108.5, -157) centre (-108.5, -158.5) ccw
  line L14 (-107, -158.5) -> (-107, -165)
  line L15 (-107, -165) -> (-13, -165)
  line L16 (-13, -165) -> (-13, -158.5)
  arc A2 (-11.5, -157) -> (-13, -158.5) centre (-11.5, -158.5) ccw
  line L17 (-11.5, -157) -> (-5, -157)
  line L18 (-5, -157) -> (-5, -13)
  line L19 (-5, -13) -> (-11.5, -13)
  arc A3 (-13, -11.5) -> (-11.5, -13) centre (-11.5, -11.5) ccw
  line L20 (-47, -165) -> (-73, -165)
  line L21 (-73, -165) -> (-47, -165)
  line L22 (-47, -165) -> (-47, -115)
  line L23 (-47, -115) -> (-73, -115)
  line L24 (-73, -115) -> (-73, -165)
  line L25 (-73, -115) -> (-47, -115)
  line L26 (-47, -115) -> (-47, -107.85)
  line L27 (-47, -107.85) -> (-73, -107.85)
  line L28 (-73, -107.85) -> (-73, -115)
  line L29 (-73, -107.85) -> (-47, -107.85)
  line L30 (-47, -107.85) -> (-47, -105)
  line L31 (-47, -105) -> (-73, -105)
  line L32 (-73, -105) -> (-73, -107.85)
  line L33 (-73, -105) -> (-68, -105)
  line L34 (-68, -105) -> (-68, -107.85)
  line L35 (-68, -107.85) -> (-73, -107.85)
  line L36 (-73, -107.85) -> (-73, -105)
  line L37 (-47, -107.85) -> (-52, -107.85)
  line L38 (-52, -107.85) -> (-52, -105)
  line L39 (-52, -105) -> (-47, -105)
  line L40 (-47, -105) -> (-47, -107.85)
  dimension "d140" = 50
  dimension "d141" = 7.15
  dimension "d142" = 5
  constraint coincident L15 L20.start
  constraint coincident L15 L20.end
  constraint horizontal L21
  constraint vertical L22
  constraint horizontal L23
  constraint vertical L24
  constraint horizontal L25
  constraint vertical L26
  constraint horizontal L27
  constraint vertical L28
  constraint horizontal L29
  constraint vertical L30
  constraint horizontal L31
  constraint vertical L32
  constraint horizontal L33
  constraint vertical L34
  constraint horizontal L35
  constraint vertical L36
  constraint coincident L27 L34.end
  constraint horizontal L37
  constraint vertical L38
  constraint horizontal L39
  constraint vertical L40
  constraint coincident L31 L38.end
  measures "d140" distance of L20.end L23.end
  measures "d141" distance of L23.end L27.end
  measures "d142" distance of L32 L34
sketch "Esquisse20" plane through (0, 5, 0) normal (0, 1, 0) x (-1, 0, 0)
  line L0 (125, -100) -> (125, -135)
  line L1 (125, -135) -> (90, -135)
  line L2 (90, -135) -> (90, -100)
  line L3 (90, -100) -> (125, -100)
  line L4 (53, -167) -> (167, -167)
  line L5 (167, -167) -> (167, -3)
  line L6 (167, -3) -> (53, -3)
  line L7 (53, -3) -> (53, -167)
  circle A0 centre (163, -7) radius 2
  circle A1 centre (57, -7) radius 2
  circle A2 centre (163, -163) radius 2
  circle A3 centre (57, -163) radius 2
  line L8 (87.5, -97.5) -> (127.5, -97.5)
  line L9 (127.5, -97.5) -> (127.5, -137.5)
  line L10 (127.5, -137.5) -> (87.5, -137.5)
  line L11 (87.5, -137.5) -> (87.5, -97.5)
  circle A4 centre (91.3, -101.3) radius 0.8
  line L12 (95.5, -102.5) -> (120, -102.5)
  line L13 (123, -105.5) -> (123, -130)
  line L14 (120, -133) -> (95.5, -133)
  line L15 (92.5, -130) -> (92.5, -105.5)
  arc A5 (95.5, -102.5) -> (92.5, -105.5) centre (95.5, -105.5) ccw
  arc A6 (123, -105.5) -> (120, -102.5) centre (120, -105.5) ccw
  arc A7 (120, -133) -> (123, -130) centre (120, -130) ccw
  arc A8 (92.5, -130) -> (95.5, -133) centre (95.5, -130) ccw
  circle A9 centre (123.7, -101.3) radius 0.8
  circle A10 centre (91.3, -133.7) radius 0.8
  circle A11 centre (123.7, -133.7) radius 0.8
  dimension "d151" = 2.5
  dimension "d152" = 2.5
  dimension "d153" = 2.5
  dimension "d154" = 3.8
  dimension "d155" = 3.8
  dimension "d156" = 3
  dimension "d159" = 32.4
  dimension "d160" = -32.4
  constraint horizontal L8
  constraint vertical L9
  constraint horizontal L10
  constraint vertical L11
  constraint horizontal L12
  constraint vertical L13
  constraint horizontal L14
  constraint vertical L15
  constraint tangent L12 A5
  constraint tangent L15 A5
  constraint tangent L12 A6
  constraint tangent L13 A6
  constraint equal A5 A6
  constraint tangent L13 A7
  constraint tangent L14 A7
  constraint equal A5 A7
  constraint tangent L14 A8
  constraint tangent L15 A8
  constraint equal A5 A8
  measures "d151" distance of L2 L11
  measures "d152" distance of L3 L8
  measures "d153" distance of L0 L9
  measures "d154" distance of L8 A4.centre
  measures "d155" distance of L11 A4.centre
  measures "d156" radius of A5
extrude "Extrusion24" add sketch "Esquisse20" against normal blind 5 contours L0 L1 L2 L3